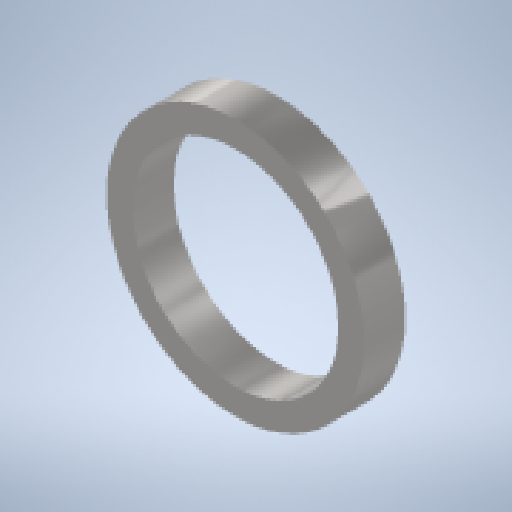
# Autodesk Inventor part: ベアリングDDA-2520
Saved by Autodesk Inventor 2024 (Build 280153000, 153)
## iProperties
Created: 2023-05-24
Part Number: ベアリングDDA-2520
Material: 鋼、炭素鋼
Document SubType Name: Modeling
Designer: yuta2
Density: 7.85 g/cm^3
Appearance: 半つや出し
Author: yuta2
Autodesk Inventor part; units mm, degrees
ref_plane "YZ Plane" through (0, 0, 0) normal (1, 0, 0) x (0, 1, 0)
ref_plane "XZ Plane" through (0, 0, 0) normal (0, 1, 0) x (-1, 0, 0)
ref_plane "XY Plane" through (0, 0, 0) normal (0, 0, 1) x (1, 0, 0)
sketch "スケッチ1" plane through (0, 0, 0) normal (1, 0, 0) x (0, 1, 0)
  line L0 (0, 0) -> (10, 0)
  line L1 (10, 0) -> (10, -4)
  line L2 (10, -4) -> (0, -4)
  line L3 (0, -4) -> (0, 0)
  line L4 (10, 0) -> (12.5, 0)
  line L5 (12.5, 0) -> (12.5, -4)
  line L6 (12.5, -4) -> (10, -4)
  line L7 (10, -4) -> (10, 0)
  dimension "d0" = 10
  dimension "d1" = 4
  dimension "d2" = 2.5
  constraints: 16 end point, 4 parallel, 2 horizontal, 2 perpendicular, 1 point on line
  measures "d0" distance of L1.end L2.end
  measures "d1" distance of L0.end L1.end
  measures "d2" distance of L5.end L6.end
revolve "回転1" add sketch "スケッチ1" angle 360 about axis through (0, 0, -4) along (0, 0, 1) contours L4 L5 L6 L1
